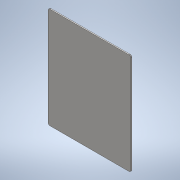
# Autodesk Inventor part: Sheet
Saved by Autodesk Inventor 2022 (Build 260153000, 153)
## iProperties
Created: 2024-10-27
Part Number: Sheet
Material: Stal, galwanizowana
Document SubType Name: Sheet Metal
Designer: NANOmatic
Density: 7.85 g/cm^3
Sheet Metal Rule: Domyślny_mm
Appearance: Galwanizowana
Author: NANOmatic
Autodesk Inventor part; units mm, degrees
ref_plane "YZ Plane" through (0, 0, 0) normal (1, 0, 0) x (0, 1, 0)
ref_plane "XZ Plane" through (0, 0, 0) normal (0, 1, 0) x (-1, 0, 0)
ref_plane "XY Plane" through (0, 0, 0) normal (0, 0, 1) x (1, 0, 0)
sketch "Szkic1" plane through (0, 0, 0) normal (0, 0, 1) x (1, 0, 0)
  line L0 (-120.5, 153.5) -> (120.5, 153.5)
  line L1 (125.5, 148.5) -> (125.5, -148.5)
  line L2 (120.5, -153.5) -> (-120.5, -153.5)
  line L3 (-125.5, -148.5) -> (-125.5, 148.5)
  line L4 (-125.5, 153.5) -> (125.5, -153.5) construction
  line L5 (125.5, 153.5) -> (-125.5, -153.5) construction
  arc A0 (-120.5, 153.5) -> (-125.5, 148.5) centre (-120.5, 148.5) ccw
  arc A1 (125.5, 148.5) -> (120.5, 153.5) centre (120.5, 148.5) ccw
  arc A2 (120.5, -153.5) -> (125.5, -148.5) centre (120.5, -148.5) ccw
  arc A3 (-125.5, -148.5) -> (-120.5, -153.5) centre (-120.5, -148.5) ccw
  point P0 (0, 0)
  dimension "d0" = 251
  dimension "d1" = 307
  dimension "d2" = 5
  measures "d0" distance of L4.end L5.end
  measures "d1" distance of L5.start L4.end
  measures "d2" radius of A0
extrude "Płyta1" add sketch "Szkic1" against normal blind 3
equation "\"d3\" = Grubość"
equation "\"PromieńGięcia\" = Grubość"
equation "\"SzerokośćGięciaPodcięcia\" = Grubość"
equation "\"GłębokośćGięciaPodcięcia\" = 0.5 * Grubość"
equation "\"RozmiarPodcięciaNarożnika\" = 4 * Grubość"
equation "\"MinimalnaPozostałość\" = 2 * Grubość"
equation "\"PromieńPrzejścia\" = PromieńGięcia"
equation "\"Rozmiar_promienia_Jacobiego\" = PromieńGięcia"
equation "\"Wielk_odstępu\" = Grubość"
equation "\"Grubość\" = 3"
